Autodesk Fusion 360 part; units mm, degrees
(part 4 of 6)
  line L297 (-107.8375, 66.9925) -> (-107.8375, 66.2921)
  arc A429 (-107.8375, 66.2921) -> (-107.7936, 66.1358) centre (-107.5375, 66.2922) ccw
  arc A430 (-108.4808, 65.4486) -> (-107.7936, 66.1358) centre (-108.2203, 65.8753) ccw
  arc A431 (-108.4808, 65.4486) -> (-108.6371, 65.4925) centre (-108.6371, 65.1928) ccw
  line L298 (-108.6371, 65.4925) -> (-109.5375, 65.4925)
  line L299 (-109.5375, 65.4925) -> (-110.4379, 65.4925)
  arc A432 (-110.4379, 65.4925) -> (-110.5942, 65.4486) centre (-110.4379, 65.1925) ccw
  circle A433 centre (-109.5375, 61.9125) radius 1.9939
  circle A434 centre (-114.6175, 61.9125) radius 0.875
  circle A435 centre (-128.27, 66.675) radius 0.875
  circle A436 centre (-133.35, 66.675) radius 1.9939
  circle A437 centre (-138.43, 66.675) radius 0.875
  circle A438 centre (-129.54, 64.135) radius 1.5
  circle A439 centre (-135.89, 61.595) radius 1.5
  arc A440 (-154.1439, 70.8983) -> (-153.4567, 70.2111) centre (-153.7172, 70.6378) ccw
  arc A441 (-154.1439, 70.8983) -> (-154.1, 71.0546) centre (-154.4, 71.0546) ccw
  line L300 (-154.1, 71.0546) -> (-154.1, 71.755)
  line L301 (-154.1, 71.755) -> (-154.1, 72.4554)
  arc A442 (-154.1, 72.4554) -> (-154.1439, 72.6117) centre (-154.4, 72.4554) ccw
  arc A443 (-153.4567, 73.2989) -> (-154.1439, 72.6117) centre (-153.7172, 72.8722) ccw
  arc A444 (-153.4567, 73.2989) -> (-153.3004, 73.255) centre (-153.3004, 73.555) ccw
  line L302 (-153.3004, 73.255) -> (-152.4, 73.255)
  line L303 (-152.4, 73.255) -> (-151.4996, 73.255)
  arc A445 (-151.4996, 73.255) -> (-151.3433, 73.2989) centre (-151.4997, 73.555) ccw
  arc A446 (-150.6561, 72.6117) -> (-151.3433, 73.2989) centre (-151.0828, 72.8722) ccw
  arc A447 (-150.6561, 72.6117) -> (-150.7, 72.4554) centre (-150.3999, 72.4553) ccw
  line L304 (-150.7, 72.4554) -> (-150.7, 71.755)
  line L305 (-150.7, 71.755) -> (-150.7, 71.0546)
  arc A448 (-150.7, 71.0546) -> (-150.6561, 70.8983) centre (-150.4, 71.0547) ccw
  arc A449 (-151.3433, 70.2111) -> (-150.6561, 70.8983) centre (-151.0828, 70.6378) ccw
  arc A450 (-151.3433, 70.2111) -> (-151.4996, 70.255) centre (-151.4996, 69.9553) ccw
  line L306 (-151.4996, 70.255) -> (-152.4, 70.255)
  line L307 (-152.4, 70.255) -> (-153.3004, 70.255)
  arc A451 (-153.3004, 70.255) -> (-153.4567, 70.2111) centre (-153.3004, 69.955) ccw
  circle A452 centre (-185.7375, 76.2) radius 1.1
  arc A453 (-173.1939, 70.8983) -> (-172.5067, 70.2111) centre (-172.7672, 70.6378) ccw
  arc A454 (-173.1939, 70.8983) -> (-173.15, 71.0546) centre (-173.45, 71.0546) ccw
  line L308 (-173.15, 71.0546) -> (-173.15, 71.755)
  line L309 (-173.15, 71.755) -> (-173.15, 72.4554)
  arc A455 (-173.15, 72.4554) -> (-173.1939, 72.6117) centre (-173.45, 72.4554) ccw
  arc A456 (-172.5067, 73.2989) -> (-173.1939, 72.6117) centre (-172.7672, 72.8722) ccw
  arc A457 (-172.5067, 73.2989) -> (-172.3504, 73.255) centre (-172.3504, 73.555) ccw
  line L310 (-172.3504, 73.255) -> (-171.45, 73.255)
  line L311 (-171.45, 73.255) -> (-170.5496, 73.255)
  arc A458 (-170.5496, 73.255) -> (-170.3933, 73.2989) centre (-170.5497, 73.555) ccw
  arc A459 (-169.7061, 72.6117) -> (-170.3933, 73.2989) centre (-170.1328, 72.8722) ccw
  arc A460 (-169.7061, 72.6117) -> (-169.75, 72.4554) centre (-169.4499, 72.4553) ccw
  line L312 (-169.75, 72.4554) -> (-169.75, 71.755)
  line L313 (-169.75, 71.755) -> (-169.75, 71.0546)
  arc A461 (-169.75, 71.0546) -> (-169.7061, 70.8983) centre (-169.45, 71.0547) ccw
  arc A462 (-170.3933, 70.2111) -> (-169.7061, 70.8983) centre (-170.1328, 70.6378) ccw
  arc A463 (-170.3933, 70.2111) -> (-170.5496, 70.255) centre (-170.5496, 69.9553) ccw
  line L314 (-170.5496, 70.255) -> (-171.45, 70.255)
  line L315 (-171.45, 70.255) -> (-172.3504, 70.255)
  arc A464 (-172.3504, 70.255) -> (-172.5067, 70.2111) centre (-172.3504, 69.955) ccw
  circle A465 centre (-147.32, 66.675) radius 0.875
  circle A466 centre (-152.4, 66.675) radius 1.9939
  circle A467 centre (-157.48, 66.675) radius 0.875
  circle A468 centre (-166.37, 66.675) radius 0.875
  circle A469 centre (-148.59, 64.135) radius 1.5
  circle A470 centre (-154.94, 61.595) radius 1.5
  circle A471 centre (-171.45, 66.675) radius 1.9939
  circle A472 centre (-176.53, 66.675) radius 0.875
  circle A473 centre (-167.64, 64.135) radius 1.5
  circle A474 centre (-173.99, 61.595) radius 1.5
  circle A475 centre (-112.0775, 56.8325) radius 1.5
  arc A476 (-122.8439, 47.0858) -> (-122.1567, 46.3986) centre (-122.4172, 46.8253) ccw
  arc A477 (-122.8439, 47.0858) -> (-122.8, 47.2421) centre (-123.1, 47.2421) ccw
  line L316 (-122.8, 47.2421) -> (-122.8, 47.9425)
  line L317 (-122.8, 47.9425) -> (-122.8, 48.6429)
  arc A478 (-122.8, 48.6429) -> (-122.8439, 48.7992) centre (-123.1, 48.6429) ccw
  arc A479 (-122.1567, 49.4864) -> (-122.8439, 48.7992) centre (-122.4172, 49.0597) ccw
  arc A480 (-122.1567, 49.4864) -> (-122.0004, 49.4425) centre (-122.0004, 49.7425) ccw
  line L318 (-122.0004, 49.4425) -> (-121.1, 49.4425)
  line L319 (-121.1, 49.4425) -> (-120.1996, 49.4425)
  arc A481 (-120.1996, 49.4425) -> (-120.0433, 49.4864) centre (-120.1997, 49.7425) ccw
  arc A482 (-119.3561, 48.7992) -> (-120.0433, 49.4864) centre (-119.7828, 49.0597) ccw
  arc A483 (-119.3561, 48.7992) -> (-119.4, 48.6429) centre (-119.0999, 48.6428) ccw
  line L320 (-119.4, 48.6429) -> (-119.4, 47.9425)
  line L321 (-119.4, 47.9425) -> (-119.4, 47.2421)
  arc A484 (-119.4, 47.2421) -> (-119.3561, 47.0858) centre (-119.1, 47.2422) ccw
  arc A485 (-120.0433, 46.3986) -> (-119.3561, 47.0858) centre (-119.7828, 46.8253) ccw
  arc A486 (-120.0433, 46.3986) -> (-120.1996, 46.4425) centre (-120.1996, 46.1428) ccw
  line L322 (-120.1996, 46.4425) -> (-121.1, 46.4425)
  line L323 (-121.1, 46.4425) -> (-122.0004, 46.4425)
  arc A487 (-122.0004, 46.4425) -> (-122.1567, 46.3986) centre (-122.0004, 46.1425) ccw
  arc A488 (-154.1439, 51.8483) -> (-153.4567, 51.1611) centre (-153.7172, 51.5878) ccw
  arc A489 (-154.1439, 51.8483) -> (-154.1, 52.0046) centre (-154.4, 52.0046) ccw
  line L324 (-154.1, 52.0046) -> (-154.1, 52.705)
  line L325 (-154.1, 52.705) -> (-154.1, 53.4054)
  arc A490 (-154.1, 53.4054) -> (-154.1439, 53.5617) centre (-154.4, 53.4054) ccw
  arc A491 (-153.4567, 54.2489) -> (-154.1439, 53.5617) centre (-153.7172, 53.8222) ccw
  arc A492 (-153.4567, 54.2489) -> (-153.3004, 54.205) centre (-153.3004, 54.505) ccw
  line L326 (-153.3004, 54.205) -> (-152.4, 54.205)
  line L327 (-152.4, 54.205) -> (-151.4996, 54.205)
  arc A493 (-151.4996, 54.205) -> (-151.3433, 54.2489) centre (-151.4997, 54.505) ccw
  arc A494 (-150.6561, 53.5617) -> (-151.3433, 54.2489) centre (-151.0828, 53.8222) ccw
  arc A495 (-150.6561, 53.5617) -> (-150.7, 53.4054) centre (-150.3999, 53.4053) ccw
  line L328 (-150.7, 53.4054) -> (-150.7, 52.705)
  line L329 (-150.7, 52.705) -> (-150.7, 52.0046)
  arc A496 (-150.7, 52.0046) -> (-150.6561, 51.8483) centre (-150.4, 52.0047) ccw
  arc A497 (-151.3433, 51.1611) -> (-150.6561, 51.8483) centre (-151.0828, 51.5878) ccw
  arc A498 (-151.3433, 51.1611) -> (-151.4996, 51.205) centre (-151.4996, 50.9053) ccw
  line L330 (-151.4996, 51.205) -> (-152.4, 51.205)
  line L331 (-152.4, 51.205) -> (-153.3004, 51.205)
  arc A499 (-153.3004, 51.205) -> (-153.4567, 51.1611) centre (-153.3004, 50.905) ccw
  circle A500 centre (-147.32, 47.625) radius 0.875
  circle A501 centre (-152.4, 47.625) radius 1.9939
  circle A502 centre (-157.48, 47.625) radius 0.875
  arc A503 (-177.9564, 47.0858) -> (-177.2692, 46.3986) centre (-177.5297, 46.8253) ccw
  arc A504 (-177.9564, 47.0858) -> (-177.9125, 47.2421) centre (-178.2125, 47.2421) ccw
  line L332 (-177.9125, 47.2421) -> (-177.9125, 47.9425)
  line L333 (-177.9125, 47.9425) -> (-177.9125, 48.6429)
  arc A505 (-177.9125, 48.6429) -> (-177.9564, 48.7992) centre (-178.2125, 48.6429) ccw
  arc A506 (-177.2692, 49.4864) -> (-177.9564, 48.7992) centre (-177.5297, 49.0597) ccw
  arc A507 (-177.2692, 49.4864) -> (-177.1129, 49.4425) centre (-177.1129, 49.7425) ccw
  line L334 (-177.1129, 49.4425) -> (-176.2125, 49.4425)
  line L335 (-176.2125, 49.4425) -> (-175.3121, 49.4425)
  arc A508 (-175.3121, 49.4425) -> (-175.1558, 49.4864) centre (-175.3122, 49.7425) ccw
  arc A509 (-174.4686, 48.7992) -> (-175.1558, 49.4864) centre (-174.8953, 49.0597) ccw
  arc A510 (-174.4686, 48.7992) -> (-174.5125, 48.6429) centre (-174.2124, 48.6428) ccw
  line L336 (-174.5125, 48.6429) -> (-174.5125, 47.9425)
  line L337 (-174.5125, 47.9425) -> (-174.5125, 47.2421)
  arc A511 (-174.5125, 47.2421) -> (-174.4686, 47.0858) centre (-174.2125, 47.2422) ccw
  arc A512 (-175.1558, 46.3986) -> (-174.4686, 47.0858) centre (-174.8953, 46.8253) ccw
  arc A513 (-175.1558, 46.3986) -> (-175.3121, 46.4425) centre (-175.3121, 46.1428) ccw
  line L338 (-175.3121, 46.4425) -> (-176.2125, 46.4425)
  line L339 (-176.2125, 46.4425) -> (-177.1129, 46.4425)
  arc A514 (-177.1129, 46.4425) -> (-177.2692, 46.3986) centre (-177.1129, 46.1425) ccw
  circle A515 centre (-33.02, 42.8625) radius 0.875
  circle A516 centre (-38.1, 42.8625) radius 1.9939
  circle A517 centre (-43.18, 42.8625) radius 0.875
  circle A518 centre (-34.29, 40.3225) radius 1.5
  circle A519 centre (-40.64, 37.7825) radius 1.5
  circle A520 centre (-52.07, 42.8625) radius 0.875
  circle A521 centre (-57.15, 42.8625) radius 1.9939
  circle A522 centre (-62.23, 42.8625) radius 0.875
  circle A523 centre (-53.34, 40.3225) radius 1.5
  circle A524 centre (-59.69, 37.7825) radius 1.5
  circle A525 centre (-71.12, 42.8625) radius 0.875
  circle A526 centre (-76.2, 42.8625) radius 1.9939
  circle A527 centre (-81.28, 42.8625) radius 0.875
  circle A528 centre (-72.39, 40.3225) radius 1.5
  circle A529 centre (-78.74, 37.7825) radius 1.5
  circle A530 centre (-90.17, 42.8625) radius 0.875
  circle A531 centre (-95.25, 42.8625) radius 1.9939
  circle A532 centre (-100.33, 42.8625) radius 0.875
  circle A533 centre (-91.44, 40.3225) radius 1.5
  circle A534 centre (-97.79, 37.7825) radius 1.5
  arc A535 (-49.3689, 28.0358) -> (-48.6817, 27.3486) centre (-48.9422, 27.7753) ccw
  arc A536 (-49.3689, 28.0358) -> (-49.325, 28.1921) centre (-49.625, 28.1921) ccw
  line L340 (-49.325, 28.1921) -> (-49.325, 28.8925)
  line L341 (-49.325, 28.8925) -> (-49.325, 29.5929)
  arc A537 (-49.325, 29.5929) -> (-49.3689, 29.7492) centre (-49.625, 29.5929) ccw
  arc A538 (-48.6817, 30.4364) -> (-49.3689, 29.7492) centre (-48.9422, 30.0097) ccw
  arc A539 (-48.6817, 30.4364) -> (-48.5254, 30.3925) centre (-48.5254, 30.6925) ccw
  line L342 (-48.5254, 30.3925) -> (-47.625, 30.3925)
  line L343 (-47.625, 30.3925) -> (-46.7246, 30.3925)
  arc A540 (-46.7246, 30.3925) -> (-46.5683, 30.4364) centre (-46.7247, 30.6925) ccw
  arc A541 (-45.8811, 29.7492) -> (-46.5683, 30.4364) centre (-46.3078, 30.0097) ccw
  arc A542 (-45.8811, 29.7492) -> (-45.925, 29.5929) centre (-45.6249, 29.5928) ccw
  line L344 (-45.925, 29.5929) -> (-45.925, 28.8925)
  line L345 (-45.925, 28.8925) -> (-45.925, 28.1921)
  arc A543 (-45.925, 28.1921) -> (-45.8811, 28.0358) centre (-45.625, 28.1922) ccw
  arc A544 (-46.5683, 27.3486) -> (-45.8811, 28.0358) centre (-46.3078, 27.7753) ccw
  arc A545 (-46.5683, 27.3486) -> (-46.7246, 27.3925) centre (-46.7246, 27.0928) ccw
  line L346 (-46.7246, 27.3925) -> (-47.625, 27.3925)
  line L347 (-47.625, 27.3925) -> (-48.5254, 27.3925)
  arc A546 (-48.5254, 27.3925) -> (-48.6817, 27.3486) centre (-48.5254, 27.0925) ccw
  circle A547 centre (-33.655, 23.8125) radius 0.875
  circle A548 centre (-42.545, 23.8125) radius 0.875
  circle A549 centre (-47.625, 23.8125) radius 1.9939
  arc A550 (-68.4189, 28.0358) -> (-67.7317, 27.3486) centre (-67.9922, 27.7753) ccw
  arc A551 (-68.4189, 28.0358) -> (-68.375, 28.1921) centre (-68.675, 28.1921) ccw
  line L348 (-68.375, 28.1921) -> (-68.375, 28.8925)
  line L349 (-68.375, 28.8925) -> (-68.375, 29.5929)
  arc A552 (-68.375, 29.5929) -> (-68.4189, 29.7492) centre (-68.675, 29.5929) ccw
  arc A553 (-67.7317, 30.4364) -> (-68.4189, 29.7492) centre (-67.9922, 30.0097) ccw
  arc A554 (-67.7317, 30.4364) -> (-67.5754, 30.3925) centre (-67.5754, 30.6925) ccw
  line L350 (-67.5754, 30.3925) -> (-66.675, 30.3925)
  line L351 (-66.675, 30.3925) -> (-65.7746, 30.3925)
  arc A555 (-65.7746, 30.3925) -> (-65.6183, 30.4364) centre (-65.7747, 30.6925) ccw
  arc A556 (-64.9311, 29.7492) -> (-65.6183, 30.4364) centre (-65.3578, 30.0097) ccw
  arc A557 (-64.9311, 29.7492) -> (-64.975, 29.5929) centre (-64.6749, 29.5928) ccw
  line L352 (-64.975, 29.5929) -> (-64.975, 28.8925)
  line L353 (-64.975, 28.8925) -> (-64.975, 28.1921)
  arc A558 (-64.975, 28.1921) -> (-64.9311, 28.0358) centre (-64.675, 28.1922) ccw
  arc A559 (-65.6183, 27.3486) -> (-64.9311, 28.0358) centre (-65.3578, 27.7753) ccw
  arc A560 (-65.6183, 27.3486) -> (-65.7746, 27.3925) centre (-65.7746, 27.0928) ccw
  line L354 (-65.7746, 27.3925) -> (-66.675, 27.3925)
  line L355 (-66.675, 27.3925) -> (-67.5754, 27.3925)
  arc A561 (-67.5754, 27.3925) -> (-67.7317, 27.3486) centre (-67.5754, 27.0925) ccw
  circle A562 centre (-52.705, 23.8125) radius 0.875
  circle A563 centre (-61.595, 23.8125) radius 0.875
  circle A564 centre (-66.675, 23.8125) radius 1.9939
  circle A565 centre (-31.115, 18.7325) radius 1.5
  circle A566 centre (-43.815, 21.2725) radius 1.5
  circle A567 centre (-50.165, 18.7325) radius 1.5
  circle A568 centre (-62.865, 21.2725) radius 1.5
  arc A569 (-87.4689, 28.0358) -> (-86.7817, 27.3486) centre (-87.0422, 27.7753) ccw
  arc A570 (-87.4689, 28.0358) -> (-87.425, 28.1921) centre (-87.725, 28.1921) ccw
  line L356 (-87.425, 28.1921) -> (-87.425, 28.8925)
  line L357 (-87.425, 28.8925) -> (-87.425, 29.5929)
  arc A571 (-87.425, 29.5929) -> (-87.4689, 29.7492) centre (-87.725, 29.5929) ccw
  arc A572 (-86.7817, 30.4364) -> (-87.4689, 29.7492) centre (-87.0422, 30.0097) ccw
  arc A573 (-86.7817, 30.4364) -> (-86.6254, 30.3925) centre (-86.6254, 30.6925) ccw
  line L358 (-86.6254, 30.3925) -> (-85.725, 30.3925)
  line L359 (-85.725, 30.3925) -> (-84.8246, 30.3925)
  arc A574 (-84.8246, 30.3925) -> (-84.6683, 30.4364) centre (-84.8247, 30.6925) ccw
  arc A575 (-83.9811, 29.7492) -> (-84.6683, 30.4364) centre (-84.4078, 30.0097) ccw
  arc A576 (-83.9811, 29.7492) -> (-84.025, 29.5929) centre (-83.7249, 29.5928) ccw
  line L360 (-84.025, 29.5929) -> (-84.025, 28.8925)
  line L361 (-84.025, 28.8925) -> (-84.025, 28.1921)
  arc A577 (-84.025, 28.1921) -> (-83.9811, 28.0358) centre (-83.725, 28.1922) ccw
  arc A578 (-84.6683, 27.3486) -> (-83.9811, 28.0358) centre (-84.4078, 27.7753) ccw
  arc A579 (-84.6683, 27.3486) -> (-84.8246, 27.3925) centre (-84.8246, 27.0928) ccw
  line L362 (-84.8246, 27.3925) -> (-85.725, 27.3925)
  line L363 (-85.725, 27.3925) -> (-86.6254, 27.3925)
  arc A580 (-86.6254, 27.3925) -> (-86.7817, 27.3486) centre (-86.6254, 27.0925) ccw
  circle A581 centre (-71.755, 23.8125) radius 0.875
  circle A582 centre (-80.645, 23.8125) radius 0.875
  circle A583 centre (-85.725, 23.8125) radius 1.9939
  arc A584 (-106.5189, 28.0358) -> (-105.8317, 27.3486) centre (-106.0922, 27.7753) ccw
  arc A585 (-106.5189, 28.0358) -> (-106.475, 28.1921) centre (-106.775, 28.1921) ccw
  line L364 (-106.475, 28.1921) -> (-106.475, 28.8925)
  line L365 (-106.475, 28.8925) -> (-106.475, 29.5929)
  arc A586 (-106.475, 29.5929) -> (-106.5189, 29.7492) centre (-106.775, 29.5929) ccw
  arc A587 (-105.8317, 30.4364) -> (-106.5189, 29.7492) centre (-106.0922, 30.0097) ccw
  arc A588 (-105.8317, 30.4364) -> (-105.6754, 30.3925) centre (-105.6754, 30.6925) ccw
  line L366 (-105.6754, 30.3925) -> (-104.775, 30.3925)
  line L367 (-104.775, 30.3925) -> (-103.8746, 30.3925)
  arc A589 (-103.8746, 30.3925) -> (-103.7183, 30.4364) centre (-103.8747, 30.6925) ccw
  arc A590 (-103.0311, 29.7492) -> (-103.7183, 30.4364) centre (-103.4578, 30.0097) ccw
  arc A591 (-103.0311, 29.7492) -> (-103.075, 29.5929) centre (-102.7749, 29.5928) ccw
  line L368 (-103.075, 29.5929) -> (-103.075, 28.8925)
  line L369 (-103.075, 28.8925) -> (-103.075, 28.1921)
  arc A592 (-103.075, 28.1921) -> (-103.0311, 28.0358) centre (-102.775, 28.1922) ccw
  arc A593 (-103.7183, 27.3486) -> (-103.0311, 28.0358) centre (-103.4578, 27.7753) ccw
  arc A594 (-103.7183, 27.3486) -> (-103.8746, 27.3925) centre (-103.8746, 27.0928) ccw
  line L370 (-103.8746, 27.3925) -> (-104.775, 27.3925)
  line L371 (-104.775, 27.3925) -> (-105.6754, 27.3925)
  arc A595 (-105.6754, 27.3925) -> (-105.8317, 27.3486) centre (-105.6754, 27.0925) ccw
  circle A596 centre (-90.805, 23.8125) radius 0.875
  circle A597 centre (-99.695, 23.8125) radius 0.875
  circle A598 centre (-104.775, 23.8125) radius 1.9939
  circle A599 centre (-69.215, 18.7325) radius 1.5
  circle A600 centre (-81.915, 21.2725) radius 1.5
  circle A601 centre (-88.265, 18.7325) radius 1.5
  circle A602 centre (-100.965, 21.2725) radius 1.5
  circle A603 centre (-107.315, 18.7325) radius 1.5
  circle A604 centre (-116.3638, 42.8625) radius 0.875
  circle A605 centre (-121.4437, 42.8625) radius 1.9939
  circle A606 centre (-126.5238, 42.8625) radius 0.875
  circle A607 centre (-117.6338, 40.3225) radius 1.5
  circle A608 centre (-123.9838, 37.7825) radius 1.5
  circle A609 centre (-148.59, 45.085) radius 1.5
  circle A610 centre (-154.94, 42.545) radius 1.5
  circle A611 centre (-171.1325, 42.8625) radius 0.875
  circle A612 centre (-176.2125, 42.8625) radius 1.9939
  circle A613 centre (-181.2925, 42.8625) radius 0.875
  circle A614 centre (-172.4025, 40.3225) radius 1.5
  circle A615 centre (-178.7525, 37.7825) radius 1.5
  circle A616 centre (-161.925, 33.3375) radius 1.1
  circle A617 centre (-109.855, 23.8125) radius 0.875
  arc A618 (-134.6746, 27.3486) -> (-133.9873, 28.0358) centre (-134.4141, 27.7753) ccw
  arc A619 (-134.6746, 27.3486) -> (-134.8309, 27.3925) centre (-134.8308, 27.0928) ccw
  line L372 (-134.8309, 27.3925) -> (-135.7312, 27.3925)
  line L373 (-135.7312, 27.3925) -> (-136.6316, 27.3925)
  arc A620 (-136.6316, 27.3925) -> (-136.7879, 27.3486) centre (-136.6316, 27.0925) ccw
  arc A621 (-137.4752, 28.0358) -> (-136.7879, 27.3486) centre (-137.0484, 27.7753) ccw
  arc A622 (-137.4752, 28.0358) -> (-137.4313, 28.1921) centre (-137.7312, 28.1921) ccw
  line L374 (-137.4312, 28.1921) -> (-137.4313, 28.8925)
  line L375 (-137.4313, 28.8925) -> (-137.4313, 29.5929)
  arc A623 (-137.4313, 29.5929) -> (-137.4752, 29.7492) centre (-137.7312, 29.5929) ccw
  arc A624 (-136.7879, 30.4364) -> (-137.4752, 29.7492) centre (-137.0484, 30.0097) ccw
  arc A625 (-136.7879, 30.4364) -> (-136.6316, 30.3925) centre (-136.6316, 30.6925) ccw
  line L376 (-136.6316, 30.3925) -> (-135.7312, 30.3925)
  line L377 (-135.7312, 30.3925) -> (-134.8309, 30.3925)
  arc A626 (-134.8309, 30.3925) -> (-134.6746, 30.4364) centre (-134.8309, 30.6925) ccw
  arc A627 (-133.9873, 29.7492) -> (-134.6746, 30.4364) centre (-134.4141, 30.0097) ccw
  arc A628 (-133.9873, 29.7492) -> (-134.0313, 29.5929) centre (-133.7312, 29.5928) ccw
  line L378 (-134.0312, 29.5929) -> (-134.0312, 28.8925)
  line L379 (-134.0312, 28.8925) -> (-134.0312, 28.1921)
  arc A629 (-134.0313, 28.1921) -> (-133.9873, 28.0358) centre (-133.7312, 28.1922) ccw
  circle A630 centre (-130.6513, 23.8125) radius 0.875
  circle A631 centre (-135.7312, 23.8125) radius 1.9939
  circle A632 centre (-140.8113, 23.8125) radius 0.875
  circle A633 centre (-131.9212, 21.2725) radius 1.5
  circle A634 centre (-138.2713, 18.7325) radius 1.5
  arc A635 (-177.9564, 28.0358) -> (-177.2692, 27.3486) centre (-177.5297, 27.7753) ccw
  arc A636 (-177.9564, 28.0358) -> (-177.9125, 28.1921) centre (-178.2125, 28.1921) ccw
  line L380 (-177.9125, 28.1921) -> (-177.9125, 28.8925)
  line L381 (-177.9125, 28.8925) -> (-177.9125, 29.5929)
  arc A637 (-177.9125, 29.5929) -> (-177.9564, 29.7492) centre (-178.2125, 29.5929) ccw
  arc A638 (-177.2692, 30.4364) -> (-177.9564, 29.7492) centre (-177.5297, 30.0097) ccw
  arc A639 (-177.2692, 30.4364) -> (-177.1129, 30.3925) centre (-177.1129, 30.6925) ccw
  line L382 (-177.1129, 30.3925) -> (-176.2125, 30.3925)
  line L383 (-176.2125, 30.3925) -> (-175.3121, 30.3925)
  arc A640 (-175.3121, 30.3925) -> (-175.1558, 30.4364) centre (-175.3122, 30.6925) ccw
  arc A641 (-174.4686, 29.7492) -> (-175.1558, 30.4364) centre (-174.8953, 30.0097) ccw
  arc A642 (-174.4686, 29.7492) -> (-174.5125, 29.5929) centre (-174.2124, 29.5928) ccw
  line L384 (-174.5125, 29.5929) -> (-174.5125, 28.8925)
  line L385 (-174.5125, 28.8925) -> (-174.5125, 28.1921)
  arc A643 (-174.5125, 28.1921) -> (-174.4686, 28.0358) centre (-174.2125, 28.1922) ccw
  arc A644 (-175.1558, 27.3486) -> (-174.4686, 28.0358) centre (-174.8953, 27.7753) ccw
  arc A645 (-175.1558, 27.3486) -> (-175.3121, 27.3925) centre (-175.3121, 27.0928) ccw
  line L386 (-175.3121, 27.3925) -> (-176.2125, 27.3925)
  line L387 (-176.2125, 27.3925) -> (-177.1129, 27.3925)
  arc A646 (-177.1129, 27.3925) -> (-177.2692, 27.3486) centre (-177.1129, 27.0925) ccw
  circle A647 centre (-171.1325, 23.8125) radius 0.875
  circle A648 centre (-176.2125, 23.8125) radius 1.9939
  circle A649 centre (-181.2925, 23.8125) radius 0.875
  circle A650 centre (-172.4025, 21.2725) radius 1.5
  circle A651 centre (-178.7525, 18.7325) radius 1.5
  circle A652 centre (-185.7375, 14.2875) radius 1.1
  arc A653 (115.3567, 8.2986) -> (116.0439, 8.9858) centre (115.6172, 8.7253) ccw
  arc A654 (115.3567, 8.2986) -> (115.2004, 8.3425) centre (115.2004, 8.0428) ccw
  line L388 (115.2004, 8.3425) -> (114.3, 8.3425)
  line L389 (114.3, 8.3425) -> (113.3996, 8.3425)
  arc A655 (113.3996, 8.3425) -> (113.2433, 8.2986) centre (113.3996, 8.0425) ccw
  arc A656 (112.5561, 8.9858) -> (113.2433, 8.2986) centre (112.9828, 8.7253) ccw
  arc A657 (112.5561, 8.9858) -> (112.6, 9.1421) centre (112.3, 9.1421) ccw
  line L390 (112.6, 9.1421) -> (112.6, 9.8425)
  line L391 (112.6, 9.8425) -> (112.6, 10.5429)
  arc A658 (112.6, 10.5429) -> (112.5561, 10.6992) centre (112.3, 10.5429) ccw
  arc A659 (113.2433, 11.3864) -> (112.5561, 10.6992) centre (112.9828, 10.9597) ccw
  arc A660 (113.2433, 11.3864) -> (113.3996, 11.3425) centre (113.3996, 11.6425) ccw
  line L392 (113.3996, 11.3425) -> (114.3, 11.3425)
  line L393 (114.3, 11.3425) -> (115.2004, 11.3425)
  arc A661 (115.2004, 11.3425) -> (115.3567, 11.3864) centre (115.2003, 11.6425) ccw
  arc A662 (116.0439, 10.6992) -> (115.3567, 11.3864) centre (115.6172, 10.9597) ccw
  arc A663 (116.0439, 10.6992) -> (116, 10.5429) centre (116.3001, 10.5428) ccw
  line L394 (116, 10.5429) -> (116, 9.8425)
  line L395 (116, 9.8425) -> (116, 9.1421)
  arc A664 (116, 9.1421) -> (116.0439, 8.9858) centre (116.3, 9.1422) ccw
  arc A665 (91.5442, 8.2986) -> (92.2314, 8.9858) centre (91.8047, 8.7253) ccw
  arc A666 (91.5442, 8.2986) -> (91.3879, 8.3425) centre (91.3879, 8.0428) ccw
  line L396 (91.3879, 8.3425) -> (90.4875, 8.3425)
  line L397 (90.4875, 8.3425) -> (89.5871, 8.3425)
  arc A667 (89.5871, 8.3425) -> (89.4308, 8.2986) centre (89.5871, 8.0425) ccw
  arc A668 (88.7436, 8.9858) -> (89.4308, 8.2986) centre (89.1703, 8.7253) ccw
  arc A669 (88.7436, 8.9858) -> (88.7875, 9.1421) centre (88.4875, 9.1421) ccw
  line L398 (88.7875, 9.1421) -> (88.7875, 9.8425)
  line L399 (88.7875, 9.8425) -> (88.7875, 10.5429)
  arc A670 (88.7875, 10.5429) -> (88.7436, 10.6992) centre (88.4875, 10.5429) ccw
  arc A671 (89.4308, 11.3864) -> (88.7436, 10.6992) centre (89.1703, 10.9597) ccw
  arc A672 (89.4308, 11.3864) -> (89.5871, 11.3425) centre (89.5871, 11.6425) ccw
  line L400 (89.5871, 11.3425) -> (90.4875, 11.3425)
  line L401 (90.4875, 11.3425) -> (91.3879, 11.3425)
  arc A673 (91.3879, 11.3425) -> (91.5442, 11.3864) centre (91.3878, 11.6425) ccw
  arc A674 (92.2314, 10.6992) -> (91.5442, 11.3864) centre (91.8047, 10.9597) ccw
  arc A675 (92.2314, 10.6992) -> (92.1875, 10.5429) centre (92.4876, 10.5428) ccw
  line L402 (92.1875, 10.5429) -> (92.1875, 9.8425)
  line L403 (92.1875, 9.8425) -> (92.1875, 9.1421)
  arc A676 (92.1875, 9.1421) -> (92.2314, 8.9858) centre (92.4875, 9.1422) ccw
  circle A677 centre (119.38, 4.7625) radius 0.875
  circle A678 centre (114.3, 4.7625) radius 1.9939
  circle A679 centre (118.11, 2.2225) radius 1.5
  circle A680 centre (111.76, -0.3175) radius 1.5
  circle A681 centre (109.22, 4.7625) radius 0.875
  circle A682 centre (95.5675, 4.7625) radius 0.875
  circle A683 centre (90.4875, 4.7625) radius 1.9939
  circle A684 centre (94.2975, 2.2225) radius 1.5
  arc A685 (72.4942, 8.2986) -> (73.1814, 8.9858) centre (72.7547, 8.7253) ccw
  arc A686 (72.4942, 8.2986) -> (72.3379, 8.3425) centre (72.3379, 8.0428) ccw
  line L404 (72.3379, 8.3425) -> (71.4375, 8.3425)
  line L405 (71.4375, 8.3425) -> (70.5371, 8.3425)
  arc A687 (70.5371, 8.3425) -> (70.3808, 8.2986) centre (70.5371, 8.0425) ccw
  arc A688 (69.6936, 8.9858) -> (70.3808, 8.2986) centre (70.1203, 8.7253) ccw
  arc A689 (69.6936, 8.9858) -> (69.7375, 9.1421) centre (69.4375, 9.1421) ccw
  line L406 (69.7375, 9.1421) -> (69.7375, 9.8425)
  line L407 (69.7375, 9.8425) -> (69.7375, 10.5429)
  arc A690 (69.7375, 10.5429) -> (69.6936, 10.6992) centre (69.4375, 10.5429) ccw
  arc A691 (70.3808, 11.3864) -> (69.6936, 10.6992) centre (70.1203, 10.9597) ccw
  arc A692 (70.3808, 11.3864) -> (70.5371, 11.3425) centre (70.5371, 11.6425) ccw
  line L408 (70.5371, 11.3425) -> (71.4375, 11.3425)
  line L409 (71.4375, 11.3425) -> (72.3379, 11.3425)
  arc A693 (72.3379, 11.3425) -> (72.4942, 11.3864) centre (72.3378, 11.6425) ccw
  arc A694 (73.1814, 10.6992) -> (72.4942, 11.3864) centre (72.7547, 10.9597) ccw
  arc A695 (73.1814, 10.6992) -> (73.1375, 10.5429) centre (73.4376, 10.5428) ccw
  line L410 (73.1375, 10.5429) -> (73.1375, 9.8425)
  line L411 (73.1375, 9.8425) -> (73.1375, 9.1421)
  arc A696 (73.1375, 9.1421) -> (73.1814, 8.9858) centre (73.4375, 9.1422) ccw
  arc A697 (53.4442, 8.2986) -> (54.1314, 8.9858) centre (53.7047, 8.7253) ccw
  arc A698 (53.4442, 8.2986) -> (53.2879, 8.3425) centre (53.2879, 8.0428) ccw
  line L412 (53.2879, 8.3425) -> (52.3875, 8.3425)
  line L413 (52.3875, 8.3425) -> (51.4871, 8.3425)
  arc A699 (51.4871, 8.3425) -> (51.3308, 8.2986) centre (51.4871, 8.0425) ccw
  arc A700 (50.6436, 8.9858) -> (51.3308, 8.2986) centre (51.0703, 8.7253) ccw
  arc A701 (50.6436, 8.9858) -> (50.6875, 9.1421) centre (50.3875, 9.1421) ccw
  line L414 (50.6875, 9.1421) -> (50.6875, 9.8425)
  line L415 (50.6875, 9.8425) -> (50.6875, 10.5429)
  arc A702 (50.6875, 10.5429) -> (50.6436, 10.6992) centre (50.3875, 10.5429) ccw
  arc A703 (51.3308, 11.3864) -> (50.6436, 10.6992) centre (51.0703, 10.9597) ccw
  arc A704 (51.3308, 11.3864) -> (51.4871, 11.3425) centre (51.4871, 11.6425) ccw
  line L416 (51.4871, 11.3425) -> (52.3875, 11.3425)
  line L417 (52.3875, 11.3425) -> (53.2879, 11.3425)
  arc A705 (53.2879, 11.3425) -> (53.4442, 11.3864) centre (53.2878, 11.6425) ccw
  arc A706 (54.1314, 10.6992) -> (53.4442, 11.3864) centre (53.7047, 10.9597) ccw
  arc A707 (54.1314, 10.6992) -> (54.0875, 10.5429) centre (54.3876, 10.5428) ccw
  line L418 (54.0875, 10.5429) -> (54.0875, 9.8425)
  line L419 (54.0875, 9.8425) -> (54.0875, 9.1421)
  arc A708 (54.0875, 9.1421) -> (54.1314, 8.9858) centre (54.3875, 9.1422) ccw
  circle A709 centre (85.4075, 4.7625) radius 0.875
  circle A710 centre (76.5175, 4.7625) radius 0.875
  circle A711 centre (71.4375, 4.7625) radius 1.9939
  circle A712 centre (75.2475, 2.2225) radius 1.5
  circle A713 centre (87.9475, -0.3175) radius 1.5
  circle A714 centre (66.3575, 4.7625) radius 0.875
  circle A715 centre (57.4675, 4.7625) radius 0.875
  circle A716 centre (52.3875, 4.7625) radius 1.9939
  circle A717 centre (56.1975, 2.2225) radius 1.5
  circle A718 centre (68.8975, -0.3175) radius 1.5
  arc A719 (120.1192, -10.7514) -> (120.8064, -10.0642) centre (120.3797, -10.3247) ccw
  arc A720 (120.1192, -10.7514) -> (119.9629, -10.7075) centre (119.9629, -11.0072) ccw
  line L420 (119.9629, -10.7075) -> (119.0625, -10.7075)
  line L421 (119.0625, -10.7075) -> (118.1621, -10.7075)
  arc A721 (118.1621, -10.7075) -> (118.0058, -10.7514) centre (118.1621, -11.0075) ccw
  arc A722 (117.3186, -10.0642) -> (118.0058, -10.7514) centre (117.7453, -10.3247) ccw
  arc A723 (117.3186, -10.0642) -> (117.3625, -9.9079) centre (117.0625, -9.9079) ccw
  line L422 (117.3625, -9.9079) -> (117.3625, -9.2075)
  line L423 (117.3625, -9.2075) -> (117.3625, -8.5071)
  arc A724 (117.3625, -8.5071) -> (117.3186, -8.3508) centre (117.0625, -8.5071) ccw
  arc A725 (118.0058, -7.6636) -> (117.3186, -8.3508) centre (117.7453, -8.0903) ccw
  arc A726 (118.0058, -7.6636) -> (118.1621, -7.7075) centre (118.1621, -7.4075) ccw
  line L424 (118.1621, -7.7075) -> (119.0625, -7.7075)
  line L425 (119.0625, -7.7075) -> (119.9629, -7.7075)
  arc A727 (119.9629, -7.7075) -> (120.1192, -7.6636) centre (119.9628, -7.4075) ccw
  arc A728 (120.8064, -8.3508) -> (120.1192, -7.6636) centre (120.3797, -8.0903) ccw
  arc A729 (120.8064, -8.3508) -> (120.7625, -8.5071) centre (121.0626, -8.5072) ccw
  line L426 (120.7625, -8.5071) -> (120.7625, -9.2075)
  line L427 (120.7625, -9.2075) -> (120.7625, -9.9079)
  arc A730 (120.7625, -9.9079) -> (120.8064, -10.0642) centre (121.0625, -9.9078) ccw
  arc A731 (101.0692, -10.7514) -> (101.7564, -10.0642) centre (101.3297, -10.3247) ccw
  arc A732 (101.0692, -10.7514) -> (100.9129, -10.7075) centre (100.9129, -11.0072) ccw
  line L428 (100.9129, -10.7075) -> (100.0125, -10.7075)
  line L429 (100.0125, -10.7075) -> (99.1121, -10.7075)
  arc A733 (99.1121, -10.7075) -> (98.9558, -10.7514) centre (99.1121, -11.0075) ccw
  arc A734 (98.2686, -10.0642) -> (98.9558, -10.7514) centre (98.6953, -10.3247) ccw
  arc A735 (98.2686, -10.0642) -> (98.3125, -9.9079) centre (98.0125, -9.9079) ccw
  line L430 (98.3125, -9.9079) -> (98.3125, -9.2075)
  line L431 (98.3125, -9.2075) -> (98.3125, -8.5071)
  arc A736 (98.3125, -8.5071) -> (98.2686, -8.3508) centre (98.0125, -8.5071) ccw
  arc A737 (98.9558, -7.6636) -> (98.2686, -8.3508) centre (98.6953, -8.0903) ccw
  arc A738 (98.9558, -7.6636) -> (99.1121, -7.7075) centre (99.1121, -7.4075) ccw
  line L432 (99.1121, -7.7075) -> (100.0125, -7.7075)
  line L433 (100.0125, -7.7075) -> (100.9129, -7.7075)
  arc A739 (100.9129, -7.7075) -> (101.0692, -7.6636) centre (100.9128, -7.4075) ccw
  arc A740 (101.7564, -8.3508) -> (101.0692, -7.6636) centre (101.3297, -8.0903) ccw
  arc A741 (101.7564, -8.3508) -> (101.7125, -8.5071) centre (102.0126, -8.5072) ccw
  line L434 (101.7125, -8.5071) -> (101.7125, -9.2075)
  line L435 (101.7125, -9.2075) -> (101.7125, -9.9079)
  arc A742 (101.7125, -9.9079) -> (101.7564, -10.0642) centre (102.0125, -9.9078) ccw
  circle A743 centre (124.1425, -14.2875) radius 0.875
  circle A744 centre (122.8725, -16.8275) radius 1.5
  circle A745 centre (119.0625, -14.2875) radius 1.9939
  circle A746 centre (113.9825, -14.2875) radius 0.875
  circle A747 centre (105.0925, -14.2875) radius 0.875
  circle A748 centre (103.8225, -16.8275) radius 1.5
  circle A749 centre (100.0125, -14.2875) radius 1.9939
  circle A750 centre (94.9325, -14.2875) radius 0.875
  arc A751 (82.0192, -10.7514) -> (82.7064, -10.0642) centre (82.2797, -10.3247) ccw
  arc A752 (82.0192, -10.7514) -> (81.8629, -10.7075) centre (81.8629, -11.0072) ccw
  line L436 (81.8629, -10.7075) -> (80.9625, -10.7075)
  line L437 (80.9625, -10.7075) -> (80.0621, -10.7075)
  arc A753 (80.0621, -10.7075) -> (79.9058, -10.7514) centre (80.0621, -11.0075) ccw
  arc A754 (79.2186, -10.0642) -> (79.9058, -10.7514) centre (79.6453, -10.3247) ccw
  arc A755 (79.2186, -10.0642) -> (79.2625, -9.9079) centre (78.9625, -9.9079) ccw
  line L438 (79.2625, -9.9079) -> (79.2625, -9.2075)
  line L439 (79.2625, -9.2075) -> (79.2625, -8.5071)
  arc A756 (79.2625, -8.5071) -> (79.2186, -8.3508) centre (78.9625, -8.5071) ccw
  arc A757 (79.9058, -7.6636) -> (79.2186, -8.3508) centre (79.6453, -8.0903) ccw
  arc A758 (79.9058, -7.6636) -> (80.0621, -7.7075) centre (80.0621, -7.4075) ccw
  line L440 (80.0621, -7.7075) -> (80.9625, -7.7075)
  line L441 (80.9625, -7.7075) -> (81.8629, -7.7075)
  arc A759 (81.8629, -7.7075) -> (82.0192, -7.6636) centre (81.8628, -7.4075) ccw
  arc A760 (82.7064, -8.3508) -> (82.0192, -7.6636) centre (82.2797, -8.0903) ccw
  arc A761 (82.7064, -8.3508) -> (82.6625, -8.5071) centre (82.9626, -8.5072) ccw
  line L442 (82.6625, -8.5071) -> (82.6625, -9.2075)
  line L443 (82.6625, -9.2075) -> (82.6625, -9.9079)
  arc A762 (82.6625, -9.9079) -> (82.7064, -10.0642) centre (82.9625, -9.9078) ccw
  arc A763 (62.9692, -10.7514) -> (63.6564, -10.0642) centre (63.2297, -10.3247) ccw
  arc A764 (62.9692, -10.7514) -> (62.8129, -10.7075) centre (62.8129, -11.0072) ccw
  line L444 (62.8129, -10.7075) -> (61.9125, -10.7075)
  line L445 (61.9125, -10.7075) -> (61.0121, -10.7075)
  arc A765 (61.0121, -10.7075) -> (60.8558, -10.7514) centre (61.0121, -11.0075) ccw
  arc A766 (60.1686, -10.0642) -> (60.8558, -10.7514) centre (60.5953, -10.3247) ccw
  arc A767 (60.1686, -10.0642) -> (60.2125, -9.9079) centre (59.9125, -9.9079) ccw
  line L446 (60.2125, -9.9079) -> (60.2125, -9.2075)
  line L447 (60.2125, -9.2075) -> (60.2125, -8.5071)
  arc A768 (60.2125, -8.5071) -> (60.1686, -8.3508) centre (59.9125, -8.5071) ccw
  arc A769 (60.8558, -7.6636) -> (60.1686, -8.3508) centre (60.5953, -8.0903) ccw
  arc A770 (60.8558, -7.6636) -> (61.0121, -7.7075) centre (61.0121, -7.4075) ccw
  line L448 (61.0121, -7.7075) -> (61.9125, -7.7075)
  line L449 (61.9125, -7.7075) -> (62.8129, -7.7075)
  arc A771 (62.8129, -7.7075) -> (62.9692, -7.6636) centre (62.8128, -7.4075) ccw
  arc A772 (63.6564, -8.3508) -> (62.9692, -7.6636) centre (63.2297, -8.0903) ccw
  arc A773 (63.6564, -8.3508) -> (63.6125, -8.5071) centre (63.9126, -8.5072) ccw
  line L450 (63.6125, -8.5071) -> (63.6125, -9.2075)
  line L451 (63.6125, -9.2075) -> (63.6125, -9.9079)
  arc A774 (63.6125, -9.9079) -> (63.6564, -10.0642) centre (63.9125, -9.9078) ccw
  circle A775 centre (86.0425, -14.2875) radius 0.875
  circle A776 centre (80.9625, -14.2875) radius 1.9939
  circle A777 centre (84.7725, -16.8275) radius 1.5
  circle A778 centre (75.8825, -14.2875) radius 0.875
  circle A779 centre (66.9925, -14.2875) radius 0.875
  circle A780 centre (61.9125, -14.2875) radius 1.9939
  circle A781 centre (65.7225, -16.8275) radius 1.5
  circle A782 centre (56.8325, -14.2875) radius 0.875
  arc A783 (34.3942, 8.2986) -> (35.0814, 8.9858) centre (34.6547, 8.7253) ccw
  arc A784 (34.3942, 8.2986) -> (34.2379, 8.3425) centre (34.2379, 8.0428) ccw
  line L452 (34.2379, 8.3425) -> (33.3375, 8.3425)
  line L453 (33.3375, 8.3425) -> (32.4371, 8.3425)
  arc A785 (32.4371, 8.3425) -> (32.2808, 8.2986) centre (32.4371, 8.0425) ccw
  arc A786 (31.5936, 8.9858) -> (32.2808, 8.2986) centre (32.0203, 8.7253) ccw
  arc A787 (31.5936, 8.9858) -> (31.6375, 9.1421) centre (31.3375, 9.1421) ccw
  line L454 (31.6375, 9.1421) -> (31.6375, 9.8425)
  line L455 (31.6375, 9.8425) -> (31.6375, 10.5429)
  arc A788 (31.6375, 10.5429) -> (31.5936, 10.6992) centre (31.3375, 10.5429) ccw
  arc A789 (32.2808, 11.3864) -> (31.5936, 10.6992) centre (32.0203, 10.9597) ccw
  arc A790 (32.2808, 11.3864) -> (32.4371, 11.3425) centre (32.4371, 11.6425) ccw
  line L456 (32.4371, 11.3425) -> (33.3375, 11.3425)
  line L457 (33.3375, 11.3425) -> (34.2379, 11.3425)
  arc A791 (34.2379, 11.3425) -> (34.3942, 11.3864) centre (34.2378, 11.6425) ccw
  arc A792 (35.0814, 10.6992) -> (34.3942, 11.3864) centre (34.6547, 10.9597) ccw
  arc A793 (35.0814, 10.6992) -> (35.0375, 10.5429) centre (35.3376, 10.5428) ccw
  line L458 (35.0375, 10.5429) -> (35.0375, 9.8425)
  line L459 (35.0375, 9.8425) -> (35.0375, 9.1421)
  arc A794 (35.0375, 9.1421) -> (35.0814, 8.9858) centre (35.3375, 9.1422) ccw
  arc A795 (15.3442, 8.2986) -> (16.0314, 8.9858) centre (15.6047, 8.7253) ccw
  arc A796 (15.3442, 8.2986) -> (15.1879, 8.3425) centre (15.1879, 8.0428) ccw
  line L460 (15.1879, 8.3425) -> (14.2875, 8.3425)
  line L461 (14.2875, 8.3425) -> (13.3871, 8.3425)
  arc A797 (13.3871, 8.3425) -> (13.2308, 8.2986) centre (13.3871, 8.0425) ccw
  arc A798 (12.5436, 8.9858) -> (13.2308, 8.2986) centre (12.9703, 8.7253) ccw
  arc A799 (12.5436, 8.9858) -> (12.5875, 9.1421) centre (12.2875, 9.1421) ccw
  line L462 (12.5875, 9.1421) -> (12.5875, 9.8425)
  line L463 (12.5875, 9.8425) -> (12.5875, 10.5429)
  arc A800 (12.5875, 10.5429) -> (12.5436, 10.6992) centre (12.2875, 10.5429) ccw
  arc A801 (13.2308, 11.3864) -> (12.5436, 10.6992) centre (12.9703, 10.9597) ccw
  arc A802 (13.2308, 11.3864) -> (13.3871, 11.3425) centre (13.3871, 11.6425) ccw
  line L464 (13.3871, 11.3425) -> (14.2875, 11.3425)
  line L465 (14.2875, 11.3425) -> (15.1879, 11.3425)
  arc A803 (15.1879, 11.3425) -> (15.3442, 11.3864) centre (15.1878, 11.6425) ccw
  arc A804 (16.0314, 10.6992) -> (15.3442, 11.3864) centre (15.6047, 10.9597) ccw
  arc A805 (16.0314, 10.6992) -> (15.9875, 10.5429) centre (16.2876, 10.5428) ccw
  line L466 (15.9875, 10.5429) -> (15.9875, 9.8425)
  line L467 (15.9875, 9.8425) -> (15.9875, 9.1421)
  arc A806 (15.9875, 9.1421) -> (16.0314, 8.9858) centre (16.2875, 9.1422) ccw
  circle A807 centre (47.3075, 4.7625) radius 0.875
  circle A808 centre (38.4175, 4.7625) radius 0.875
  circle A809 centre (33.3375, 4.7625) radius 1.9939
  circle A810 centre (37.1475, 2.2225) radius 1.5
  circle A811 centre (49.8475, -0.3175) radius 1.5
  circle A812 centre (30.7975, -0.3175) radius 1.5
  circle A813 centre (28.2575, 4.7625) radius 0.875
  circle A814 centre (19.3675, 4.7625) radius 0.875
  circle A815 centre (14.2875, 4.7625) radius 1.9939
  circle A816 centre (18.0975, 2.2225) radius 1.5
  circle A817 centre (11.7475, -0.3175) radius 1.5
  arc A818 (-6.5064, 8.9858) -> (-5.8192, 8.2986) centre (-6.0797, 8.7253) ccw
  arc A819 (-6.5064, 8.9858) -> (-6.4625, 9.1421) centre (-6.7625, 9.1421) ccw
  line L468 (-6.4625, 9.1421) -> (-6.4625, 9.8425)
  line L469 (-6.4625, 9.8425) -> (-6.4625, 10.5429)
  arc A820 (-6.4625, 10.5429) -> (-6.5064, 10.6992) centre (-6.7625, 10.5429) ccw
  arc A821 (-5.8192, 11.3864) -> (-6.5064, 10.6992) centre (-6.0797, 10.9597) ccw
  arc A822 (-5.8192, 11.3864) -> (-5.6629, 11.3425) centre (-5.6629, 11.6425) ccw
  line L470 (-5.6629, 11.3425) -> (-4.7625, 11.3425)
  line L471 (-4.7625, 11.3425) -> (-3.8621, 11.3425)
  arc A823 (-3.8621, 11.3425) -> (-3.7058, 11.3864) centre (-3.8622, 11.6425) ccw
  arc A824 (-3.0186, 10.6992) -> (-3.7058, 11.3864) centre (-3.4453, 10.9597) ccw
  arc A825 (-3.0186, 10.6992) -> (-3.0625, 10.5429) centre (-2.7624, 10.5428) ccw
  line L472 (-3.0625, 10.5429) -> (-3.0625, 9.8425)
  line L473 (-3.0625, 9.8425) -> (-3.0625, 9.1421)
  arc A826 (-3.0625, 9.1421) -> (-3.0186, 8.9858) centre (-2.7625, 9.1422) ccw
  arc A827 (-3.7058, 8.2986) -> (-3.0186, 8.9858) centre (-3.4453, 8.7253) ccw
  arc A828 (-3.7058, 8.2986) -> (-3.8621, 8.3425) centre (-3.8621, 8.0428) ccw
  line L474 (-3.8621, 8.3425) -> (-4.7625, 8.3425)
  line L475 (-4.7625, 8.3425) -> (-5.6629, 8.3425)
  arc A829 (-5.6629, 8.3425) -> (-5.8192, 8.2986) centre (-5.6629, 8.0425) ccw
  arc A830 (-25.5564, 8.9858) -> (-24.8692, 8.2986) centre (-25.1297, 8.7253) ccw
  arc A831 (-25.5564, 8.9858) -> (-25.5125, 9.1421) centre (-25.8125, 9.1421) ccw
  line L476 (-25.5125, 9.1421) -> (-25.5125, 9.8425)
  line L477 (-25.5125, 9.8425) -> (-25.5125, 10.5429)
  arc A832 (-25.5125, 10.5429) -> (-25.5564, 10.6992) centre (-25.8125, 10.5429) ccw
  arc A833 (-24.8692, 11.3864) -> (-25.5564, 10.6992) centre (-25.1297, 10.9597) ccw
  arc A834 (-24.8692, 11.3864) -> (-24.7129, 11.3425) centre (-24.7129, 11.6425) ccw
  line L478 (-24.7129, 11.3425) -> (-23.8125, 11.3425)
  line L479 (-23.8125, 11.3425) -> (-22.9121, 11.3425)
  arc A835 (-22.9121, 11.3425) -> (-22.7558, 11.3864) centre (-22.9122, 11.6425) ccw
  arc A836 (-22.0686, 10.6992) -> (-22.7558, 11.3864) centre (-22.4953, 10.9597) ccw
  arc A837 (-22.0686, 10.6992) -> (-22.1125, 10.5429) centre (-21.8124, 10.5428) ccw
  line L480 (-22.1125, 10.5429) -> (-22.1125, 9.8425)
  line L481 (-22.1125, 9.8425) -> (-22.1125, 9.1421)
  arc A838 (-22.1125, 9.1421) -> (-22.0686, 8.9858) centre (-21.8125, 9.1422) ccw
  arc A839 (-22.7558, 8.2986) -> (-22.0686, 8.9858) centre (-22.4953, 8.7253) ccw
  arc A840 (-22.7558, 8.2986) -> (-22.9121, 8.3425) centre (-22.9121, 8.0428) ccw
  line L482 (-22.9121, 8.3425) -> (-23.8125, 8.3425)
  line L483 (-23.8125, 8.3425) -> (-24.7129, 8.3425)
  arc A841 (-24.7129, 8.3425) -> (-24.8692, 8.2986) centre (-24.7129, 8.0425) ccw
  circle A842 centre (9.2075, 4.7625) radius 0.875
  circle A843 centre (0.3175, 4.7625) radius 0.875
  circle A844 centre (-4.7625, 4.7625) radius 1.9939
  circle A845 centre (-0.9525, 2.2225) radius 1.5
  circle A846 centre (-7.3025, -0.3175) radius 1.5
  circle A847 centre (-9.8425, 4.7625) radius 0.875
  circle A848 centre (-18.7325, 4.7625) radius 0.875
  circle A849 centre (-23.8125, 4.7625) radius 1.9939
  circle A850 centre (-20.0025, 2.2225) radius 1.5
  circle A851 centre (-26.3525, -0.3175) radius 1.5
  arc A852 (43.9192, -10.7514) -> (44.6064, -10.0642) centre (44.1797, -10.3247) ccw
  arc A853 (43.9192, -10.7514) -> (43.7629, -10.7075) centre (43.7629, -11.0072) ccw
  line L484 (43.7629, -10.7075) -> (42.8625, -10.7075)
  line L485 (42.8625, -10.7075) -> (41.9621, -10.7075)
  arc A854 (41.9621, -10.7075) -> (41.8058, -10.7514) centre (41.9621, -11.0075) ccw
  arc A855 (41.1186, -10.0642) -> (41.8058, -10.7514) centre (41.5453, -10.3247) ccw
  arc A856 (41.1186, -10.0642) -> (41.1625, -9.9079) centre (40.8625, -9.9079) ccw
  line L486 (41.1625, -9.9079) -> (41.1625, -9.2075)
  line L487 (41.1625, -9.2075) -> (41.1625, -8.5071)
  arc A857 (41.1625, -8.5071) -> (41.1186, -8.3508) centre (40.8625, -8.5071) ccw
  arc A858 (41.8058, -7.6636) -> (41.1186, -8.3508) centre (41.5453, -8.0903) ccw
  arc A859 (41.8058, -7.6636) -> (41.9621, -7.7075) centre (41.9621, -7.4075) ccw
  line L488 (41.9621, -7.7075) -> (42.8625, -7.7075)
  line L489 (42.8625, -7.7075) -> (43.7629, -7.7075)
  arc A860 (43.7629, -7.7075) -> (43.9192, -7.6636) centre (43.7628, -7.4075) ccw
  arc A861 (44.6064, -8.3508) -> (43.9192, -7.6636) centre (44.1797, -8.0903) ccw
  arc A862 (44.6064, -8.3508) -> (44.5625, -8.5071) centre (44.8626, -8.5072) ccw
  line L490 (44.5625, -8.5071) -> (44.5625, -9.2075)
  line L491 (44.5625, -9.2075) -> (44.5625, -9.9079)
  arc A863 (44.5625, -9.9079) -> (44.6064, -10.0642) centre (44.8625, -9.9078) ccw
  arc A864 (24.8692, -10.7514) -> (25.5564, -10.0642) centre (25.1297, -10.3247) ccw
  arc A865 (24.8692, -10.7514) -> (24.7129, -10.7075) centre (24.7129, -11.0072) ccw
  line L492 (24.7129, -10.7075) -> (23.8125, -10.7075)
  line L493 (23.8125, -10.7075) -> (22.9121, -10.7075)
  arc A866 (22.9121, -10.7075) -> (22.7558, -10.7514) centre (22.9121, -11.0075) ccw
  arc A867 (22.0686, -10.0642) -> (22.7558, -10.7514) centre (22.4953, -10.3247) ccw
  arc A868 (22.0686, -10.0642) -> (22.1125, -9.9079) centre (21.8125, -9.9079) ccw
  line L494 (22.1125, -9.9079) -> (22.1125, -9.2075)
  line L495 (22.1125, -9.2075) -> (22.1125, -8.5071)
  arc A869 (22.1125, -8.5071) -> (22.0686, -8.3508) centre (21.8125, -8.5071) ccw
  arc A870 (22.7558, -7.6636) -> (22.0686, -8.3508) centre (22.4953, -8.0903) ccw
  arc A871 (22.7558, -7.6636) -> (22.9121, -7.7075) centre (22.9121, -7.4075) ccw
  line L496 (22.9121, -7.7075) -> (23.8125, -7.7075)
  line L497 (23.8125, -7.7075) -> (24.7129, -7.7075)
  arc A872 (24.7129, -7.7075) -> (24.8692, -7.6636) centre (24.7128, -7.4075) ccw
  arc A873 (25.5564, -8.3508) -> (24.8692, -7.6636) centre (25.1297, -8.0903) ccw
  arc A874 (25.5564, -8.3508) -> (25.5125, -8.5071) centre (25.8126, -8.5072) ccw
  line L498 (25.5125, -8.5071) -> (25.5125, -9.2075)
  line L499 (25.5125, -9.2075) -> (25.5125, -9.9079)
  arc A875 (25.5125, -9.9079) -> (25.5564, -10.0642) centre (25.8125, -9.9078) ccw
  circle A876 centre (47.9425, -14.2875) radius 0.875
  circle A877 centre (42.8625, -14.2875) radius 1.9939
  circle A878 centre (46.6725, -16.8275) radius 1.5
  circle A879 centre (37.7825, -14.2875) radius 0.875
  circle A880 centre (28.8925, -14.2875) radius 0.875
  circle A881 centre (23.8125, -14.2875) radius 1.9939
  circle A882 centre (27.6225, -16.8275) radius 1.5
  circle A883 centre (18.7325, -14.2875) radius 0.875
  arc A884 (5.8192, -10.7514) -> (6.5064, -10.0642) centre (6.0797, -10.3247) ccw
  arc A885 (5.8192, -10.7514) -> (5.6629, -10.7075) centre (5.6629, -11.0072) ccw
  line L500 (5.6629, -10.7075) -> (4.7625, -10.7075)
  line L501 (4.7625, -10.7075) -> (3.8621, -10.7075)
  arc A886 (3.8621, -10.7075) -> (3.7058, -10.7514) centre (3.8621, -11.0075) ccw
  arc A887 (3.0186, -10.0642) -> (3.7058, -10.7514) centre (3.4453, -10.3247) ccw
  arc A888 (3.0186, -10.0642) -> (3.0625, -9.9079) centre (2.7625, -9.9079) ccw
  line L502 (3.0625, -9.9079) -> (3.0625, -9.2075)
  line L503 (3.0625, -9.2075) -> (3.0625, -8.5071)
  arc A889 (3.0625, -8.5071) -> (3.0186, -8.3508) centre (2.7625, -8.5071) ccw
  arc A890 (3.7058, -7.6636) -> (3.0186, -8.3508) centre (3.4453, -8.0903) ccw
  arc A891 (3.7058, -7.6636) -> (3.8621, -7.7075) centre (3.8621, -7.4075) ccw
  line L504 (3.8621, -7.7075) -> (4.7625, -7.7075)
  line L505 (4.7625, -7.7075) -> (5.6629, -7.7075)
  arc A892 (5.6629, -7.7075) -> (5.8192, -7.6636) centre (5.6628, -7.4075) ccw
  arc A893 (6.5064, -8.3508) -> (5.8192, -7.6636) centre (6.0797, -8.0903) ccw
  arc A894 (6.5064, -8.3508) -> (6.4625, -8.5071) centre (6.7626, -8.5072) ccw
  line L506 (6.4625, -8.5071) -> (6.4625, -9.2075)
  line L507 (6.4625, -9.2075) -> (6.4625, -9.9079)
  arc A895 (6.4625, -9.9079) -> (6.5064, -10.0642) centre (6.7625, -9.9078) ccw
  arc A896 (-16.0314, -10.0642) -> (-15.3442, -10.7514) centre (-15.6047, -10.3247) ccw
  arc A897 (-16.0314, -10.0642) -> (-15.9875, -9.9079) centre (-16.2875, -9.9079) ccw
  line L508 (-15.9875, -9.9079) -> (-15.9875, -9.2075)
  line L509 (-15.9875, -9.2075) -> (-15.9875, -8.5071)
  arc A898 (-15.9875, -8.5071) -> (-16.0314, -8.3508) centre (-16.2875, -8.5071) ccw
  arc A899 (-15.3442, -7.6636) -> (-16.0314, -8.3508) centre (-15.6047, -8.0903) ccw
  arc A900 (-15.3442, -7.6636) -> (-15.1879, -7.7075) centre (-15.1879, -7.4075) ccw
  line L510 (-15.1879, -7.7075) -> (-14.2875, -7.7075)
  line L511 (-14.2875, -7.7075) -> (-13.3871, -7.7075)
  arc A901 (-13.3871, -7.7075) -> (-13.2308, -7.6636) centre (-13.3872, -7.4075) ccw
  arc A902 (-12.5436, -8.3508) -> (-13.2308, -7.6636) centre (-12.9703, -8.0903) ccw
  arc A903 (-12.5436, -8.3508) -> (-12.5875, -8.5071) centre (-12.2874, -8.5072) ccw
  line L512 (-12.5875, -8.5071) -> (-12.5875, -9.2075)
  line L513 (-12.5875, -9.2075) -> (-12.5875, -9.9079)
  arc A904 (-12.5875, -9.9079) -> (-12.5436, -10.0642) centre (-12.2875, -9.9078) ccw
  arc A905 (-13.2308, -10.7514) -> (-12.5436, -10.0642) centre (-12.9703, -10.3247) ccw
  arc A906 (-13.2308, -10.7514) -> (-13.3871, -10.7075) centre (-13.3871, -11.0072) ccw
  line L514 (-13.3871, -10.7075) -> (-14.2875, -10.7075)
  line L515 (-14.2875, -10.7075) -> (-15.1879, -10.7075)
  arc A907 (-15.1879, -10.7075) -> (-15.3442, -10.7514) centre (-15.1879, -11.0075) ccw
  circle A908 centre (9.8425, -14.2875) radius 0.875
  circle A909 centre (4.7625, -14.2875) radius 1.9939
  circle A910 centre (8.5725, -16.8275) radius 1.5
  circle A911 centre (-0.3175, -14.2875) radius 0.875
  circle A912 centre (-9.2075, -14.2875) radius 0.875
  circle A913 centre (-14.2875, -14.2875) radius 1.9939
  circle A914 centre (-10.4775, -16.8275) radius 1.5
  circle A915 centre (-19.3675, -14.2875) radius 0.875
  circle A916 centre (-28.2575, -14.2875) radius 0.875
  circle A917 centre (116.5225, -19.3675) radius 1.5
  circle A918 centre (97.4725, -19.3675) radius 1.5
  arc A919 (120.1192, -34.5639) -> (120.8064, -33.8767) centre (120.3797, -34.1372) ccw
  arc A920 (120.1192, -34.5639) -> (119.9629, -34.52) centre (119.9629, -34.8197) ccw
  line L516 (119.9629, -34.52) -> (119.0625, -34.52)
  line L517 (119.0625, -34.52) -> (118.1621, -34.52)
  arc A921 (118.1621, -34.52) -> (118.0058, -34.5639) centre (118.1621, -34.82) ccw
  arc A922 (117.3186, -33.8767) -> (118.0058, -34.5639) centre (117.7453, -34.1372) ccw
  arc A923 (117.3186, -33.8767) -> (117.3625, -33.7204) centre (117.0625, -33.7204) ccw
  line L518 (117.3625, -33.7204) -> (117.3625, -33.02)
  line L519 (117.3625, -33.02) -> (117.3625, -32.3196)
  arc A924 (117.3625, -32.3196) -> (117.3186, -32.1633) centre (117.0625, -32.3196) ccw
  arc A925 (118.0058, -31.4761) -> (117.3186, -32.1633) centre (117.7453, -31.9028) ccw
  arc A926 (118.0058, -31.4761) -> (118.1621, -31.52) centre (118.1621, -31.22) ccw
  line L520 (118.1621, -31.52) -> (119.0625, -31.52)
  line L521 (119.0625, -31.52) -> (119.9629, -31.52)
  arc A927 (119.9629, -31.52) -> (120.1192, -31.4761) centre (119.9628, -31.22) ccw
  arc A928 (120.8064, -32.1633) -> (120.1192, -31.4761) centre (120.3797, -31.9028) ccw
  arc A929 (120.8064, -32.1633) -> (120.7625, -32.3196) centre (121.0626, -32.3197) ccw
  line L522 (120.7625, -32.3196) -> (120.7625, -33.02)
  line L523 (120.7625, -33.02) -> (120.7625, -33.7204)
  arc A930 (120.7625, -33.7204) -> (120.8064, -33.8767) centre (121.0625, -33.7203) ccw
  circle A931 centre (107.1563, -26.1938) radius 1.1
  arc A932 (96.3067, -34.5639) -> (96.9939, -33.8767) centre (96.5672, -34.1372) ccw
  arc A933 (96.3067, -34.5639) -> (96.1504, -34.52) centre (96.1504, -34.8197) ccw
  line L524 (96.1504, -34.52) -> (95.25, -34.52)
  line L525 (95.25, -34.52) -> (94.3496, -34.52)
  arc A934 (94.3496, -34.52) -> (94.1933, -34.5639) centre (94.3496, -34.82) ccw
  arc A935 (93.5061, -33.8767) -> (94.1933, -34.5639) centre (93.9328, -34.1372) ccw
  arc A936 (93.5061, -33.8767) -> (93.55, -33.7204) centre (93.25, -33.7204) ccw
  line L526 (93.55, -33.7204) -> (93.55, -33.02)
  line L527 (93.55, -33.02) -> (93.55, -32.3196)